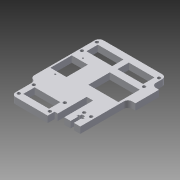
# Autodesk Inventor part: yCarBottom
Saved by Autodesk Inventor 2013 (Build 170138000, 138)
## iProperties
Created: 2015-01-14
Part Number: yCarBottom
Material: Generic
Document SubType Name: Modeling
Designer: dzban
Density: 1 g/cm^3
Author: dzban
Autodesk Inventor part; units mm, degrees
ref_plane "YZ Plane" through (0, 0, 0) normal (1, 0, 0) x (0, 1, 0)
ref_plane "XZ Plane" through (0, 0, 0) normal (0, 1, 0) x (-1, 0, 0)
ref_plane "XY Plane" through (0, 0, 0) normal (0, 0, 1) x (1, 0, 0)
sketch "Sketch1" plane through (0, 0, 0) normal (0, 0, 1) x (1, 0, 0)
  line L0 (-30, 44) -> (-30, 64)
  line L1 (-30, 64) -> (-2, 64)
  line L2 (-2, 64) -> (-2, 44)
  line L3 (-2, 44) -> (-30, 44)
  line L4 (-61.5, 40) -> (-61.5, 60)
  line L5 (-61.5, 60) -> (-46.5, 60)
  line L6 (-46.5, 60) -> (-46.5, 40)
  line L7 (-46.5, 40) -> (-61.5, 40)
  line L8 (-53, 6.2) -> (-53, 16.8)
  line L9 (-53, 16.8) -> (-29, 16.8)
  line L10 (-29, 16.8) -> (-29, 6.2)
  line L11 (-29, 6.2) -> (-53, 6.2)
  line L12 (-29, 70.2) -> (-29, 80.8)
  line L13 (-29, 80.8) -> (-5, 80.8)
  line L14 (-5, 80.8) -> (-5, 70.2)
  line L15 (-5, 70.2) -> (-29, 70.2)
  line L16 (-58, 70.2) -> (-58, 80.8)
  line L17 (-58, 80.8) -> (-34, 80.8)
  line L18 (-34, 80.8) -> (-34, 70.2)
  line L19 (-34, 70.2) -> (-58, 70.2)
  circle A0 centre (-3, 19.5) radius 1.5
  circle A1 centre (-9.5, 19.5) radius 1.5
  circle A2 centre (-26.5, 18.5) radius 1.5
  circle A3 centre (-26.5, 4.5) radius 1.5
  circle A4 centre (-55.5, 4.5) radius 1.5
  circle A5 centre (-55.5, 18.5) radius 1.5
  circle A6 centre (-2.5, 68.5) radius 1.5
  circle A7 centre (-60.5, 68.5) radius 1.5
  circle A8 centre (-60.5, 82.5) radius 1.5
  circle A9 centre (-2.5, 82.5) radius 1.5
  circle A10 centre (-54, 37) radius 0.75
  circle A11 centre (-54, 63) radius 0.75
  arc A12 (-63, 26.3448) -> (-60.5004, 22.6368) centre (-59, 26.3448) ccw
  arc A13 (-58.0008, 18.9289) -> (-60.5004, 22.6368) centre (-62.0008, 18.9289) ccw
  line L20 (-58.0008, 18.9289) -> (-58.0008, 4)
  arc A14 (-58.0008, 4) -> (-54.0008, 0) centre (-54.0008, 4) ccw
  line L21 (-54.0008, 0) -> (-24, 0)
  line L22 (-24, 0) -> (-24, 6.4)
  line L23 (-24, 6.4) -> (-21, 6.4)
  line L24 (-21, 6.4) -> (-21, 33.4)
  line L25 (-21, 33.4) -> (-15, 33.4)
  line L26 (-15, 33.4) -> (-15, 6.4)
  line L27 (-15, 6.4) -> (-9, 6.4)
  line L28 (-9, 6.4) -> (-9, 13.4)
  line L29 (-9, 13.4) -> (-10.25, 13.4)
  line L30 (-10.25, 13.4) -> (-10.25, 15.2)
  line L31 (-10.25, 15.2) -> (-9, 15.2)
  line L32 (-9, 15.2) -> (-9, 17)
  line L33 (-9, 17) -> (-6, 17)
  line L34 (-6, 17) -> (-6, 15.2)
  line L35 (-6, 15.2) -> (-4.75, 15.2)
  line L36 (-4.75, 15.2) -> (-4.75, 13.4)
  line L37 (-4.75, 13.4) -> (-6, 13.4)
  line L38 (-6, 13.4) -> (-6, 6.4)
  line L39 (-6, 6.4) -> (0, 6.4)
  line L40 (0, 6.4) -> (0, 47)
  arc A15 (4, 51) -> (0, 47) centre (4, 47) ccw
  line L41 (7, 51) -> (4, 51)
  line L42 (7, 73) -> (7, 51)
  line L43 (4, 73) -> (7, 73)
  arc A16 (0, 77) -> (4, 73) centre (4, 77) ccw
  line L44 (0, 77) -> (0, 83)
  arc A17 (0, 83) -> (-4, 87) centre (-4, 83) ccw
  line L45 (-4, 87) -> (-59, 87)
  arc A18 (-59, 87) -> (-63, 83) centre (-59, 83) ccw
  line L46 (-63, 83) -> (-63, 26.3448)
  point P0 (0, 0)
  point P1 (0, 0)
  constraints: 94 end point, 19 centre point, 14 point on circle
extrude "Extrusion1" add sketch "Sketch1" along normal blind 6
body "Solid1"
